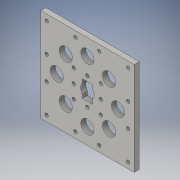
# Autodesk Inventor part: Top
Saved by Autodesk Inventor 2016 (Build 200138000, 138)
## iProperties
Created: 2015-07-01
Part Number: Top
Material: Generic
Document SubType Name: Modeling
Designer: Rodrigo
Density: 1 g/cm^3
Appearance: Default
Author: Rodrigo
Autodesk Inventor part; units mm, degrees
ref_plane "YZ Plane" through (0, 0, 0) normal (1, 0, 0) x (0, 1, 0)
ref_plane "XZ Plane" through (0, 0, 0) normal (0, 1, 0) x (-1, 0, 0)
ref_plane "XY Plane" through (0, 0, 0) normal (0, 0, 1) x (1, 0, 0)
sketch "Sketch1" plane through (0, 0, 0) normal (0, 0, 1) x (1, 0, 0)
  circle A0 centre (12.7279, -12.7279) radius 3.895 projected
  circle A1 centre (0, -18) radius 3.895 projected
  circle A2 centre (-12.7279, -12.7279) radius 3.895 projected
  circle A3 centre (-18, 0) radius 3.895 projected
  circle A4 centre (-12.7279, 12.7279) radius 3.895 projected
  circle A5 centre (0, 18) radius 3.895 projected
  circle A6 centre (12.7279, 12.7279) radius 3.895 projected
  circle A7 centre (18, 0) radius 3.895 projected
  circle A8 centre (8, 0) radius 1 projected
  circle A9 centre (8, -8) radius 1
  circle A10 centre (0, -8) radius 1 projected
  circle A11 centre (-8, -8) radius 1
  circle A12 centre (-8, 0) radius 1 projected
  circle A13 centre (-8, 8) radius 1
  circle A14 centre (0, 8) radius 1 projected
  circle A15 centre (8, 8) radius 1
  arc A16 (3, -2.6458) -> (3, 2.6458) centre (0, 0) ccw projected
  line L0 (3, -2.6458) -> (3, -5) projected
  line L1 (3, -5) -> (-3, -5) projected
  line L2 (-3, -5) -> (-3, -2.6458) projected
  arc A17 (-3, 2.6458) -> (-3, -2.6458) centre (0, 0) ccw projected
  line L3 (-3, 2.6458) -> (-3, 5) projected
  line L4 (-3, 5) -> (3, 5) projected
  line L5 (3, 5) -> (3, 2.6458) projected
  circle A18 centre (-24, -24) radius 1 projected
  circle A19 centre (-7, 24) radius 1 projected
  circle A20 centre (7, 24) radius 1 projected
  line L6 (27.5, -27.5) -> (-27.5, -27.5)
  line L7 (-27.5, -27.5) -> (-27.5, 27.5)
  line L8 (-27.5, 27.5) -> (27.5, 27.5)
  line L9 (27.5, 27.5) -> (27.5, -27.5)
  line L10 (27.5, -27.5) -> (-27.5, 27.5) construction
  line L11 (-27.5, -27.5) -> (27.5, 27.5) construction
  circle A21 centre (-24, 7) radius 1
  circle A22 centre (-24, -7) radius 1
  circle A23 centre (24, 24) radius 1
  circle A24 centre (7, -24) radius 1
  circle A25 centre (-7, -24) radius 1
  circle A26 centre (24, 7) radius 1
  circle A27 centre (24, -7) radius 1
  line L12 (0, -27.5) -> (0, 27.5) construction
  circle A28 centre (24, -24) radius 1
  circle A29 centre (-24, 24) radius 1
  point P0 (0, 0)
  dimension "d0" = 55
  dimension "d1" = 55
  dimension "d6" = 2
  dimension "d7" = 2
  dimension "d8" = 2
  dimension "d9" = 2
  constraints: 14 end point, 9 symmetric about line, 4 centre point, 4 midpoint, 2 parallel, 1 horizontal, 1 perpendicular, 9 other
  measures "d0" distance of L7.end L8.end
  measures "d1" distance of L6.end L7.end
  measures "d6" diameter of A13
  measures "d7" diameter of A15
  measures "d8" diameter of A9
  measures "d9" diameter of A11
extrude "Extrusion2" add sketch "Sketch1" along normal blind 3
equation "\"d7\" = d6"
equation "\"d8\" = d6"
equation "\"d9\" = d6"
body "Solid2"
